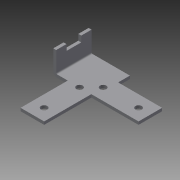
# Autodesk Inventor part: Gusset Connector 2
Saved by Autodesk Inventor 2013 (Build 170138000, 138)
## iProperties
Created: 2013-02-01
Part Number: Gusset Connector 2
Material: Generic
Document SubType Name: Sheet Metal
Designer: actoennies
Density: 1 g/cm^3
Sheet Metal Rule: Default
Mass: 9.78659 g
Surface Area: 74.0209 cm^2
Volume: 9.78659 cm^3
Author: actoennies
Autodesk Inventor part; units mm, degrees
ref_plane "YZ Plane" through (0, 0, 0) normal (1, 0, 0) x (0, 1, 0)
ref_plane "XZ Plane" through (0, 0, 0) normal (0, 1, 0) x (-1, 0, 0)
ref_plane "XY Plane" through (0, 0, 0) normal (0, 0, 1) x (1, 0, 0)
sketch "Sketch1" plane through (0, 0, 0) normal (0, 1, 0) x (-1, 0, 0)
  circle A0 centre (-63.5, 12.7) radius 3.3782
  circle A1 centre (-25.4, 12.7) radius 3.3782
  circle A2 centre (-12.7, 25.4) radius 3.3782
  circle A3 centre (-12.7, 63.5) radius 3.3782
  line L0 (0, 76.2) -> (0, 25.4)
  line L1 (-25.4, 76.2) -> (0, 76.2)
  line L2 (-25.4, 25.4) -> (-25.4, 76.2)
  line L3 (-76.2, 25.4) -> (-25.4, 25.4)
  line L4 (-76.2, 0) -> (-76.2, 25.4)
  line L5 (-28.829, 0) -> (-76.2, 0)
  line L6 (15.621, -25.4) -> (-28.829, -25.4)
  line L7 (-28.829, -25.4) -> (-28.829, 0)
  line L8 (0, 25.4) -> (15.621, 25.4)
  line L9 (15.621, 25.4) -> (15.621, -25.4)
  line L10 (15.621, -25.4) -> (15.621, -25.4)
  point P0 (0, 0)
  point P1 (0, 0)
  dimension "d32" = 15.621
  dimension "d44" = 50.8
  measures "d32" distance of L0.end L8.end
  measures "d44" distance of L8.end L9.end
extrude "Plate1" add sketch "Sketch1" along normal blind 3.175
sketch "Sketch7" plane through (0, 0, 0) normal (0, -1, 0) x (1, 0, 0)
  line L0 (28.829, -25.4) -> (-15.621, -25.4) projected
  line L1 (28.829, 0) -> (28.829, -25.4) projected
  line L2 (76.2, 0) -> (28.829, 0) projected
  line L3 (-15.621, 25.4) -> (0, 25.4) projected
  line L4 (0, 25.4) -> (0, 0)
  line L5 (0, 0) -> (28.829, 0)
  line L6 (-15.621, -25.4) -> (-15.621, 25.4)
  constraints: 6 end point, 2 perpendicular, 1 collinear
extrude "Cut3" cut sketch "Sketch7" against normal blind 3.175
equation "\"d45\" = Thickness"
equation "\"BendRadius\" = Thickness"
equation "\"BendReliefWidth\" = Thickness"
equation "\"BendReliefDepth\" = 0.5 * Thickness"
equation "\"CornerReliefSize\" = 4 * Thickness"
equation "\"MinimumRemnant\" = 2 * Thickness"
equation "\"TransitionRadius\" = BendRadius"
equation "\"JacobiRadiusSize\" = BendRadius"
equation "\"GapSize\" = Thickness"
equation "\"d1\" = BendRadius"
equation "\"Thickness\" = 3.175"
body "Solid1"
